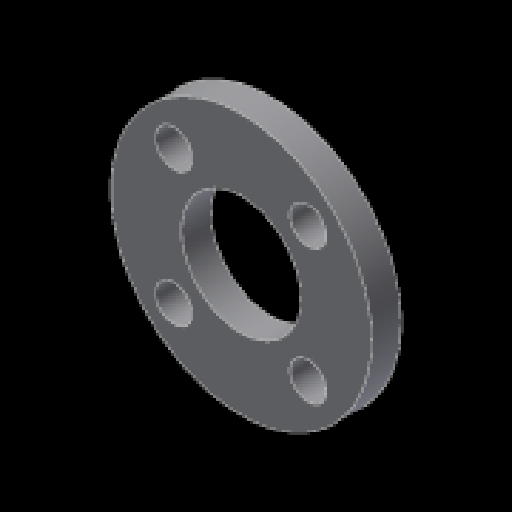
# Autodesk Inventor part: WheelEncoderMagnetAlignmentFlange
Saved by Autodesk Inventor 2025.2 (Build 292293000, 293)
## iProperties
Created: 2026-02-08
Part Number: WheelEncoderMagnetAlignmentFlange
Material: Generic
Document SubType Name: Sheet Metal
Designer: valer
Density: 1 g/cm^3
Sheet Metal Rule: Default_mm
Appearance: Default
Author: valer
Autodesk Inventor part; units mm, degrees
ref_plane "YZ Plane" through (0, 0, 0) normal (1, 0, 0) x (0, 1, 0)
ref_plane "XZ Plane" through (0, 0, 0) normal (0, 1, 0) x (-1, 0, 0)
ref_plane "XY Plane" through (0, 0, 0) normal (0, 0, 1) x (1, 0, 0)
sketch "Base" plane through (0, 0, 0) normal (0, 0, 1) x (1, 0, 0)
  circle A0 centre (0, 0) radius 3.9873
  circle A1 centre (0, 0) radius 8.7406
  line L0 (-4.5, -4.5) -> (4.5, -4.5) construction
  line L1 (4.5, -4.5) -> (4.5, 4.5) construction
  line L2 (4.5, 4.5) -> (-4.5, 4.5) construction
  line L3 (-4.5, 4.5) -> (-4.5, -4.5) construction
  line L4 (-4.5, -4.5) -> (4.5, 4.5) construction
  line L5 (4.5, -4.5) -> (-4.5, 4.5) construction
  line L6 (-12.2369, 0) -> (12.2369, 0) construction
  circle A2 centre (0, 0) radius 6.364 construction
  circle A3 centre (-4.5, 4.5) radius 1.225
  circle A4 centre (4.5, 4.5) radius 1.225
  circle A5 centre (4.5, -4.5) radius 1.225
  circle A6 centre (-4.5, -4.5) radius 1.225
  dimension "d0" = 7.9746
  dimension "d1" = 4.7533
  dimension "d2" = 2.3767
  dimension "d3" = 2.45
  dimension "d4" = 9
  measures "d0" diameter of A0
  measures "d1" radial gap between concentric circles of A1 A0
  measures "d3" diameter of A3
  measures "d4" distance of L1.end L2.end
extrude "Plate1" add sketch "Base" along normal blind 2
equation "\"d2\" = 0.5 * d1"
equation "\"d7\" = Thickness"
equation "\"BendRadius\" = Thickness"
equation "\"BendReliefWidth\" = Thickness"
equation "\"BendReliefDepth\" = 0.5 * Thickness"
equation "\"CornerReliefSize\" = 4 * Thickness"
equation "\"MinimumRemnant\" = 2 * Thickness"
equation "\"TransitionRadius\" = BendRadius"
equation "\"JacobiRadiusSize\" = BendRadius"
equation "\"GapSize\" = Thickness"
equation "\"Thickness\" = 2"
body "Solid2"
